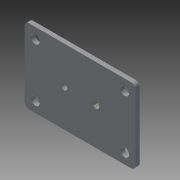
# Autodesk Inventor part: frontcncld
Saved by Autodesk Inventor 2014 (Build 180170000, 170)
## iProperties
Created: 2013-06-04
Part Number: frontcncld
Material: Generisch
Document SubType Name: Modeling
Designer: Felix
Density: 1 g/cm^3
Appearance: Vorgabe
Author: Felix
Autodesk Inventor part; units mm, degrees
ref_plane "YZ Plane" through (0, 0, 0) normal (1, 0, 0) x (0, 1, 0)
ref_plane "XZ Plane" through (0, 0, 0) normal (0, 1, 0) x (-1, 0, 0)
ref_plane "XY Plane" through (0, 0, 0) normal (0, 0, 1) x (1, 0, 0)
sketch "Skizze2" plane through (0, 0, 0) normal (0, 1, 0) x (-1, 0, 0)
  line L0 (0, 0) -> (52, 0)
  line L1 (52, 0) -> (52, 35)
  line L2 (52, 35) -> (0, 35)
  line L3 (0, 35) -> (0, 0)
  dimension "d3" = 52
  dimension "d4" = 35
  constraints: 8 end point, 2 parallel, 1 horizontal, 1 perpendicular
  measures "d3" distance of L1.end L2.end
  measures "d4" distance of L0.end L1.end
extrude "Extrusion1" add sketch "Skizze2" along normal blind 2
sketch "Skizze3" plane through (0, 0, 0) normal (0, -1, 0) x (1, 0, 0)
  line L0 (0, 35) -> (0, 0) projected
  line L1 (-52, 0) -> (-52, 35) projected
  line L2 (-52, 17.5) -> (0, 17.5)
  line L3 (-33.5, 17.5) -> (-18.5, 17.5)
  line L4 (-33.5, 17.5) -> (-52, 17.5)
  line L5 (-18.5, 17.5) -> (0, 17.5)
  circle A0 centre (-33.5, 17.5) radius 1.525
  circle A1 centre (-18.5, 17.5) radius 1.525
  dimension "d7" = 15
  dimension "d8" = 3.05
  dimension "d9" = 3.05
  constraints: 8 end point, 3 collinear, 2 centre point, 2 coincident, 2 midpoint, 2 point on line
  measures "d7" distance of L3.start L3.end
  measures "d8" diameter of A0
  measures "d9" diameter of A1
extrude "Extrusion2" cut sketch "Skizze3" against normal through all
sketch "Skizze6" plane through (0, 0, 0) normal (0, -1, 0) x (1, 0, 0)
  line L0 (0, 0) -> (-52, 0) projected
  line L1 (0, 35) -> (0, 0) projected
  line L2 (-52, 35) -> (0, 35) projected
  line L3 (-52, 0) -> (-52, 35) projected
  line L4 (-47, 30) -> (-5, 30)
  line L5 (-5, 30) -> (-5, 5)
  line L6 (-5, 5) -> (-47, 5)
  line L7 (-47, 5) -> (-47, 30)
  dimension "d17" = 5
  dimension "d18" = 5
  dimension "d19" = 5
  dimension "d20" = 5
  constraints: 8 end point, 2 parallel, 1 horizontal, 1 perpendicular
  measures "d17" distance between parallel lines of L7 L3
  measures "d18" distance between parallel lines of L5 L1
  measures "d19" distance between parallel lines of L2 L4
  measures "d20" distance between parallel lines of L6 L0
hole "Bohrung1" at (-5, 0, 5) at (-5, 0, 30) at (-47, 0, 30) at (-47, 0, 5) direction (0, 1, 0) diameter 4.1 end through all
fillet "Rundung2" radius 2 4 edges at (-52, 1, 35) (-52, 1, 0) (0, 1, 0) (0, 1, 35)
